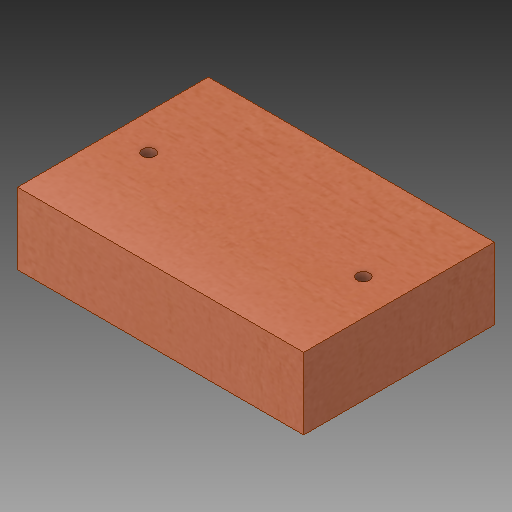
# Autodesk Inventor part: WoodHandRail
Saved by Autodesk Inventor 2019.3 (Build 233278000, 278)
## iProperties
Created: 2019-04-05
Part Number: WoodHandRail
Material: Wood (Walnut)
Document SubType Name: Modeling
Designer: steele
Density: 0.55 g/cm^3
Appearance: Walnut - Natural Polished
Author: steele
Autodesk Inventor part; units mm, degrees
ref_plane "YZ Plane" through (0, 0, 0) normal (1, 0, 0) x (0, 1, 0)
ref_plane "XZ Plane" through (0, 0, 0) normal (0, 1, 0) x (-1, 0, 0)
ref_plane "XY Plane" through (0, 0, 0) normal (0, 0, 1) x (1, 0, 0)
sketch "Sketch1" plane through (0, 0, 0) normal (0, 1, 0) x (-1, 0, 0)
  line L0 (76.2, 50.8) -> (-76.2, 50.8)
  line L1 (-76.2, 50.8) -> (-76.2, -50.8)
  line L2 (-76.2, -50.8) -> (76.2, -50.8)
  line L3 (76.2, -50.8) -> (76.2, 50.8)
  line L4 (76.2, 50.8) -> (-76.2, -50.8) construction
  line L5 (-76.2, 50.8) -> (76.2, -50.8) construction
  point P0 (0, 0)
  dimension "d0" = 152.4
  dimension "d1" = 101.6
  constraints: 12 end point, 2 midpoint, 2 parallel, 1 horizontal, 1 perpendicular
  measures "d0" distance of L0.start L0.end
  measures "d1" distance of L2.end L0.start
extrude "Extrusion1" add sketch "Sketch1" against normal blind 38.1
sketch "Sketch2" plane through (0, 0, 0) normal (0, 1, 0) x (1, 0, 0)
  point P0 (-57.15, 0)
  point P1 (57.15, 0)
hole "Hole1" at (-57.15, 0, 0) at (57.15, 0, 0) direction (0, -1, 0) diameter 6.7564 depth 38.1
body "Solid1"
